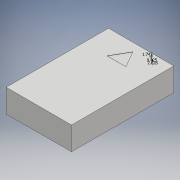
# Autodesk Inventor part: battery model
Saved by Autodesk Inventor 2017 (Build 210142000, 142)
## iProperties
Created: 2017-05-03
Part Number: battery model
Material: Generic
Document SubType Name: Modeling
Designer: caleb
Density: 1 g/cm^3
Appearance: Default
Author: caleb
Autodesk Inventor part; units mm, degrees
ref_plane "YZ Plane" through (0, 0, 0) normal (1, 0, 0) x (0, 1, 0)
ref_plane "XZ Plane" through (0, 0, 0) normal (0, 1, 0) x (-1, 0, 0)
ref_plane "XY Plane" through (0, 0, 0) normal (0, 0, 1) x (1, 0, 0)
sketch "Sketch1" plane through (0, 0, 0) normal (0, 0, 1) x (1, 0, 0)
  line L0 (0, 0) -> (34.5, 0)
  line L1 (34.5, 0) -> (34.5, 54)
  line L2 (34.5, 54) -> (0, 54)
  line L3 (0, 54) -> (0, 0)
  dimension "d0" = 54
  dimension "d1" = 34.5
  constraints: 8 end point, 2 parallel, 1 horizontal, 1 perpendicular
  measures "d0" distance of L2.end L0.start
  measures "d1" distance of L0.start L0.end
extrude "Extrusion1" add sketch "Sketch1" along normal blind 12.25
sketch "Sketch2" plane through (0, 0, 12.25) normal (0, 0, 1) x (1, 0, 0)
  line L0 (12.25, 41) -> (17.25, 49.6603)
  line L1 (17.25, 49.6603) -> (22.25, 41)
  line L2 (22.25, 41) -> (12.25, 41)
  line L3 (0, 0) -> (34.5, 0) construction
  point P0 (17.25, 41)
  point P1 (17.25, 0)
  dimension "d4" = 41
  dimension "d5" = 10
  constraints: 6 end point, 2 equal length, 2 midpoint, 1 horizontal, 1 vertical alignment
  measures "d4" distance from line of L3 L0.start
  measures "d5" distance of L1.end L0.start
extrude "Extrusion2" cut sketch "Sketch2" against normal blind 0.1
sketch "Sketch3" plane through (0, 54, 0) normal (0, 1, 0) x (1, 0, 0)
  line L0 (34.5, 0) -> (0, 0) construction
  line L1 (0, 0) -> (0, -12.25) construction
  line L2 (34.5, -12.25) -> (0, -12.25) construction
  line L3 (34.5, 0) -> (34.5, -12.25) construction
  line L4 (4, 0) -> (4, -3)
  line L5 (4, -3) -> (0, -3)
  line L6 (4, 0) -> (0, 0)
  line L7 (0, -3) -> (0, 0)
  point P0 (0, 0)
  dimension "d8" = 3
  dimension "d9" = 4
  constraints: 8 end point, 2 collinear, 2 point on line, 1 perpendicular, 1 vertical
  measures "d8" distance of L4.start L4.end
  measures "d9" distance of L4.end L5.end
extrude "Extrusion3" cut sketch "Sketch3" against normal blind 3
sketch "Sketch4" plane through (0, 54, 12.25) normal (0, 1, 0) x (1, 0, 0)
  line L0 (4, 12.25) -> (4, 9.25) projected
  line L1 (4, 9.25) -> (0, 9.25) projected
  line L2 (0, 9.25) -> (0, 0) projected
  line L3 (34.5, 0) -> (0, 0) projected
  line L4 (34.5, 12.25) -> (34.5, 0) projected
  line L5 (34.5, 12.25) -> (4, 12.25) projected
  line L6 (6, 10.1) -> (10, 10.1)
  line L7 (10, 10.1) -> (10, 5.2)
  line L8 (10, 5.2) -> (6, 5.2)
  line L9 (6, 5.2) -> (6, 10.1)
  line L10 (12.6, 10.1) -> (16.6, 10.1)
  line L11 (16.6, 10.1) -> (16.6, 5.2)
  line L12 (16.6, 5.2) -> (12.6, 5.2)
  line L13 (12.6, 5.2) -> (12.6, 10.1)
  line L14 (19.2, 10.1) -> (23.2, 10.1)
  line L15 (23.2, 10.1) -> (23.2, 5.2)
  line L16 (23.2, 5.2) -> (19.2, 5.2)
  line L17 (19.2, 5.2) -> (19.2, 10.1)
  line L18 (10, 10.1) -> (12.6, 10.1) construction
  line L19 (2, 4.16) -> (4.43, 4.16)
  line L20 (4.43, 4.16) -> (4.43, 8.8603)
  line L21 (4.43, 8.8603) -> (2, 8.8603)
  line L22 (2, 8.8603) -> (2, 4.16)
  point P0 (0, 12.25)
  dimension "d12" = 2.15
  dimension "d13" = 4.9
  dimension "d14" = 6
  dimension "d15" = 4
  dimension "d16" = 12.6
  dimension "d17" = 2.6
  dimension "d18" = 2.6
  dimension "d21" = 2
  dimension "d22" = 4.7003
  dimension "d23" = 2.43
  dimension "d24" = 4.16
  constraints: 34 end point, 8 parallel, 4 horizontal, 4 perpendicular, 4 point on line, 3 collinear
  measures "d12" distance between parallel lines of L5 L6
  measures "d13" distance of L8.end L6.start
  measures "d14" distance between parallel lines of L9 L2
  measures "d15" distance of L7.end L8.end
  measures "d16" distance between parallel lines of L2 L13
  measures "d17" distance of L6.end L10.start
  measures "d18" distance of L14.start L10.end
  measures "d21" distance between parallel lines of L2 L22
  measures "d22" distance of L21.end L19.start
  measures "d23" distance of L19.start L19.end
  measures "d24" distance between parallel lines of L3 L19
extrude "Extrusion4" cut sketch "Sketch4" against normal blind 0.9 contours L6 L7 L8 L9 | L10 L11 L12 L13 | L14 L15 L16 L17
sketch "Sketch5" plane through (0, 54, 12.25) normal (0, 1, 0) x (1, 0, 0)
  line L0 (20.3264, 2.5717) -> (22.0736, 2.5717) construction
  line L1 (22.0736, 2.5717) -> (22.0736, 2.1463) construction
  line L2 (22.0736, 2.1463) -> (20.3264, 2.1463) construction
  line L3 (20.3264, 2.1463) -> (20.3264, 2.5717) construction
  line L4 (23.2, 5.2) -> (19.2, 5.2) projected
  line L5 (15.4736, 2.1463) -> (13.7264, 2.1463) construction
  line L6 (13.7264, 2.1463) -> (13.7264, 2.5717) construction
  line L7 (13.7264, 2.5717) -> (15.4736, 2.5717) construction
  line L8 (15.4736, 2.5717) -> (15.4736, 2.1463) construction
  line L9 (16.6, 5.2) -> (12.6, 5.2) projected
  line L10 (8.8736, 2.5717) -> (8.8736, 2.1463) construction
  line L11 (8.8736, 2.1463) -> (7.1264, 2.1463) construction
  line L12 (7.1264, 2.1463) -> (7.1264, 2.5717) construction
  line L13 (7.1264, 2.5717) -> (8.8736, 2.5717) construction
  line L14 (10, 5.2) -> (6, 5.2) projected
  point P0 (0, 12.25)
  point P1 (21.2, 5.2)
  point P2 (21.2, 2.5717)
  point P3 (14.6, 2.1463)
  point P4 (14.6, 5.2)
  point P5 (8, 2.1463)
  point P6 (8, 5.2)
  point P7 (20.3264, 2.359)
  point P8 (15.4736, 2.359)
  point P9 (8.8736, 2.359)
  dimension "d25" = 2.6283
  dimension "d26" = 1.7472
  dimension "d27" = 0.4254
  constraints: 9 midpoint, 4 collinear, 3 vertical alignment, 2 horizontal, 2 horizontal alignment, 6 other
  measures "d25" distance between parallel lines of L0 L4
  measures "d26" distance of L1.end L2.end
  measures "d27" distance of L0.end L1.end
equation "\"d18\" = d17"
body "Solid1"
